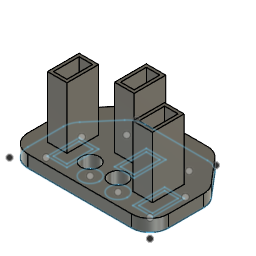
iec blank (Autodesk Fusion 360 design; units mm, degrees)
Autodesk Fusion 360 part; units mm, degrees
sketch "Sketch1" plane through (0, 0, 0) normal (0, 0, 1) x (1, 0, 0)
  line L0 (25.75, 36.6) -> (42.75, 36.6)
  line L1 (40.15, 44.6) -> (42.35, 44.6)
  line L2 (42.35, 44.6) -> (42.35, 40.4)
  line L3 (42.35, 40.4) -> (40.15, 40.4)
  line L4 (40.15, 40.4) -> (40.15, 44.6)
  line L5 (26.15, 40.4) -> (26.15, 44.6)
  line L6 (28.35, 44.6) -> (28.35, 40.4)
  line L7 (26.15, 44.6) -> (28.35, 44.6)
  line L8 (26.15, 40.4) -> (28.35, 40.4)
  line L9 (33.15, 48.6) -> (35.35, 48.6)
  line L10 (35.35, 48.6) -> (35.35, 44.4)
  line L11 (35.35, 44.4) -> (33.15, 44.4)
  line L12 (33.15, 44.4) -> (33.15, 48.6)
  line L13 (29.1351, 52.4) -> (39.36, 52.4)
  line L14 (22.75, 39.6) -> (22.75, 45.4272)
  line L15 (45.75, 39.6) -> (45.75, 45.3997)
  arc A0 (22.75, 39.6) -> (25.75, 36.6) centre (25.75, 39.6) ccw
  arc A1 (42.75, 36.6) -> (45.75, 39.6) centre (42.75, 39.6) ccw
  circle A2 centre (36.5318, 40.5854) radius 1.5
  circle A3 centre (31.9682, 40.5854) radius 1.5
  line L16 (23.4665, 47.3729) -> (26.8517, 51.3457)
  line L17 (45.0387, 47.3393) -> (41.6487, 51.3396)
  arc A4 (23.4665, 47.3729) -> (22.75, 45.4272) centre (25.75, 45.4272) ccw
  arc A5 (29.1351, 52.4) -> (26.8517, 51.3457) centre (29.1351, 49.4) ccw
  arc A6 (41.6487, 51.3396) -> (39.36, 52.4) centre (39.36, 49.4) ccw
  arc A7 (45.75, 45.3997) -> (45.0387, 47.3393) centre (42.75, 45.3997) ccw
  line L18 (28.85, 45.1) -> (28.85, 39.9)
  line L19 (25.65, 39.9) -> (28.85, 39.9)
  line L20 (25.65, 39.9) -> (25.65, 45.1)
  line L21 (25.65, 45.1) -> (28.85, 45.1)
  line L22 (35.85, 49.1) -> (35.85, 43.9)
  line L23 (35.85, 43.9) -> (32.65, 43.9)
  line L24 (32.65, 43.9) -> (32.65, 49.1)
  line L25 (32.65, 49.1) -> (35.85, 49.1)
  line L26 (42.85, 45.1) -> (42.85, 39.9)
  line L27 (42.85, 39.9) -> (39.65, 39.9)
  line L28 (39.65, 39.9) -> (39.65, 45.1)
  line L29 (39.65, 45.1) -> (42.85, 45.1)
  point P0 (22.75, 36.6)
  point P1 (45.75, 36.6)
  point P2 (27.75, 52.4)
  point P3 (40.75, 52.4)
  dimension "d1" = 23
  dimension "d22" = 13
  dimension "d29" = 3
  dimension "d31" = 3
  dimension "d32" = 3
  dimension "d34" = 3
  dimension "d35" = -0.5
  dimension "d36" = -0.5
  dimension "d37" = -0.5
  constraint horizontal L0
  constraint horizontal L1
  constraint vertical L2
  constraint horizontal L3
  constraint vertical L4
  constraint vertical L6
  constraint vertical L5
  constraint perpendicular L5 L8
  constraint horizontal L9
  constraint vertical L10
  constraint horizontal L11
  constraint vertical L12
  constraint horizontal L13
  constraint perpendicular L0 L14
  constraint perpendicular L0 L15
  constraint coincident P0 L0
  constraint coincident P0 L14
  constraint tangent L0 A0
  constraint tangent L14 A0
  constraint coincident P1 L0
  constraint coincident P1 L15
  constraint tangent L0 A1
  constraint tangent L15 A1
  constraint equal A0 A1
  constraint coincident P2 L13
  constraint coincident P3 L13
  constraint tangent L14 A4
  constraint tangent L16 A4
  constraint tangent L13 A5
  constraint tangent L16 A5
  constraint equal A4 A5
  constraint tangent L13 A6
  constraint tangent L17 A6
  constraint equal A4 A6
  constraint tangent L17 A7
  constraint tangent L15 A7
  constraint equal A4 A7
  measures "d1" distance of P0 P1
  measures "d22" distance of P2 P3
  measures "d29" radius of A0
  measures "d31" diameter of A2
  measures "d32" diameter of A3
  measures "d34" radius of A4
extrude "Extrude1" add sketch "Sketch1" along normal blind 2 makes body 1 at (26.8833, 41.8, 0) makes body 2 at (33.8833, 47.2, 0) makes body 3 at (29.4506, 48.5152, 0) makes body 4 at (40.8833, 41.8, 0)
extrude "Extrude2" add sketch "Sketch1" along normal blind 11 contours L18 L19 L20 L21 | L22 L23 L24 L25 | L26 L27 L28 L29 bodies 1 2 3 4
extrude "Extrude5" add 1 faces at (25.8167, 43.2, 11) along direction (0, 0, 1) blind 1 on bodies 1 bodies 1
extrude "Extrude6" add 1 faces at (32.8167, 47.2, 11) along direction (0, 0, 1) blind 1 on bodies 1 bodies 1
extrude "Extrude7" add 1 faces at (42.6833, 41.8, 11) along direction (0, 0, 1) blind 1 on bodies 1 bodies 1
extrude "Extrude10" cut 1 faces at (33.8833, 47.2, 2) along direction (0, 0, -1) blind 1 on bodies 1 bodies 1
extrude "Extrude8" [suppressed]
extrude "Extrude3" [suppressed]
